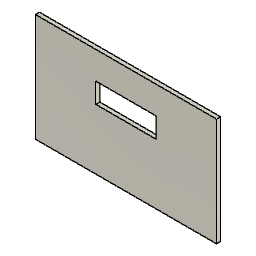
unsorted_smarties_back_panel (Autodesk Fusion 360 design; units mm, degrees)
Autodesk Fusion 360 part; units mm, degrees
sketch "Unsorted Smarties Back" plane through (0, 0, 0) normal (0, 1, 0) x (1, 0, 0)
  line L0 (0, 0) -> (270, 0)
  line L1 (270, 0) -> (270, -161)
  line L2 (270, -161) -> (0, -161)
  line L3 (0, -161) -> (0, 0)
  dimension "d1" = 270
  dimension "d2" = 161
  constraint horizontal L0
  constraint vertical L1
  constraint horizontal L2
  constraint vertical L3
  constraint coincident L0.start L3.end
  measures "d1" distance of L0.start L0.end
  measures "d2" distance of L0.end L1.end
extrude "Extrude1" add sketch "Unsorted Smarties Back" along normal blind 6
sketch "Smartie Feed" plane through (0, 0, 0) normal (0, -1, 0) x (1, 0, 0)
  line L0 (270, 161) -> (0, 161)
  line L1 (0, 161) -> (0, 0)
  line L2 (0, 0) -> (270, 0)
  line L3 (270, 0) -> (270, 161)
  line L4 (90, 120) -> (180, 120)
  line L5 (180, 120) -> (180, 90)
  line L6 (180, 90) -> (90, 90)
  line L7 (90, 90) -> (90, 120)
  dimension "d6" = 90
  dimension "d7" = 90
  dimension "d8" = 41
  dimension "d9" = 30
  dimension "d12" = 90
  constraint horizontal L4
  constraint vertical L5
  constraint horizontal L6
  constraint vertical L7
  measures "d6" distance of L1 L7
  measures "d7" distance of L3 L5
  measures "d8" distance of L0 L4
  measures "d9" distance of L4.end L5.end
  measures "d12" distance of L5 L7
extrude "Extrude2" cut sketch "Smartie Feed" against normal blind 6 contours L4 L5 L6 L7
equation "mdfThickness = 6 mm" comment "Thickness of the MDF fibre board"
equation "d4 = mdfThickness"
equation "d10 = -mdfThickness"
named bodies: "Unsorted Smarties Back Panel"
